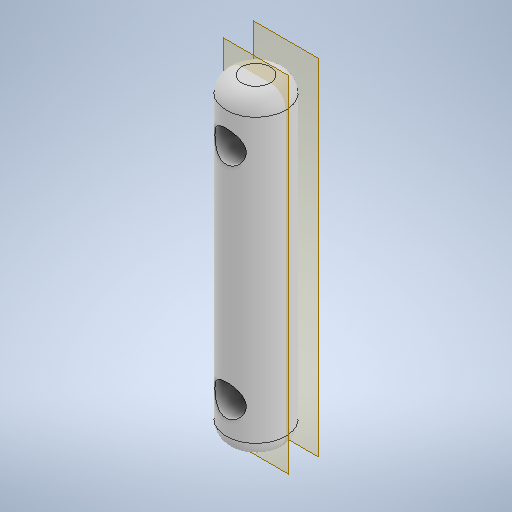
# Autodesk Inventor part: Part2
Saved by Autodesk Inventor 2025.2 (Build 292293000, 293)
## iProperties
Created: 2025-04-11
Part Number: Part2
Material: Generic
Document SubType Name: Sheet Metal
Designer: ziyuz
Density: 1 g/cm^3
Sheet Metal Rule: Default_mm
Appearance: Default
Author: ziyuz
Autodesk Inventor part; units mm, degrees
ref_plane "YZ Plane" through (0, 0, 0) normal (1, 0, 0) x (0, 1, 0)
ref_plane "XZ Plane" through (0, 0, 0) normal (0, 1, 0) x (-1, 0, 0)
sketch "Sketch1" plane through (0, 0, 0) normal (0, 1, 0) x (-1, 0, 0)
  circle A0 centre (0, 0) radius 9.5
  dimension "d0" = 19
  constraints: 1 centre point, 1 coincident
  measures "d0" diameter of A0
extrude "Extrusion1" add sketch "Sketch1" along normal blind 100
ref_plane "Work Plane1" through (0, 0, -9.5) normal (0, 0, 1) x (1, 0, 0)
sketch "Sketch2" plane through (0, 0, -9.5) normal (0, 0, 1) x (1, 0, 0)
  line L0 (0, 0) -> (0, 100)
  line L1 (9.5, 100) -> (-9.5, 100) projected
  line L2 (0, 50) -> (0, 15)
  line L3 (0, 50) -> (0, 85)
  circle A0 centre (0, 15) radius 5
  circle A1 centre (0, 85) radius 5
  dimension "d4" = 35
  dimension "d5" = 35
  dimension "d6" = 10
  dimension "d7" = 10
  constraints: 6 end point, 2 centre point, 2 coincident, 2 midpoint, 2 point on line
  measures "d4" distance of L2.start L2.end
  measures "d5" distance of L2.start L3.end
  measures "d6" diameter of A0
  measures "d7" diameter of A1
extrude "Extrusion2" cut sketch "Sketch2" along normal blind 20
fillet "Fillet1" radius 5 2 edges at (9.5, 100, 0) (9.5, 0, 0)
equation "\"BendRadius\" = Thickness"
equation "\"BendReliefWidth\" = Thickness"
equation "\"BendReliefDepth\" = 0.5 * Thickness"
equation "\"CornerReliefSize\" = 4 * Thickness"
equation "\"MinimumRemnant\" = 2 * Thickness"
equation "\"TransitionRadius\" = BendRadius"
equation "\"JacobiRadiusSize\" = BendRadius"
equation "\"GapSize\" = Thickness"
equation "\"Thickness\" = 0.5"
body "Solid1"
